Autodesk Fusion 360 part; units mm, degrees
note: some values were not read from the file. Set by a fixed rule: which sketch regions a step uses.
(part 4 of 59)
  spline S16 degree 5 poles (20.11, 33.4575) (20.11, 33.4576) (20.1102, 33.4577) (20.1104, 33.458) (20.1107, 33.4583) (20.1112, 33.4589) (20.1118, 33.4595) (20.1125, 33.4602) (20.1132, 33.461) (20.114, 33.4619) (20.1149, 33.4629) (20.1159, 33.4639) (20.1169, 33.4651) (20.118, 33.4663) (20.1192, 33.4675) (20.1204, 33.4689) (20.1217, 33.4704) (20.123, 33.4719) (20.1245, 33.4735) (20.126, 33.4752) (20.1275, 33.4769) (20.1291, 33.4787) (20.1308, 33.4806) (20.1325, 33.4826) (20.1343, 33.4847) (20.1361, 33.4868) (20.138, 33.489) (20.1399, 33.4912) (20.1419, 33.4936) (20.144, 33.496) (20.1461, 33.4984) (20.1482, 33.501) (20.1504, 33.5036) (20.1527, 33.5063) (20.155, 33.509) (20.1573, 33.5119) (20.1597, 33.5148) (20.1622, 33.5177) (20.1647, 33.5207) (20.1672, 33.5238) (20.1698, 33.527) (20.1724, 33.5302) (20.1751, 33.5335) (20.1778, 33.5368) (20.1806, 33.5403) (20.1834, 33.5437) (20.1862, 33.5473) (20.1891, 33.5509) (20.192, 33.5546) (20.195, 33.5583) (20.198, 33.5621) (20.201, 33.566) (20.2041, 33.5699) (20.2072, 33.5739) (20.2103, 33.5779) (20.2135, 33.582) (20.2167, 33.5862) (20.22, 33.5904) (20.2233, 33.5947) (20.2266, 33.599) (20.23, 33.6034) (20.2333, 33.6079) (20.2368, 33.6124) (20.2402, 33.617) (20.2437, 33.6216) (20.2472, 33.6263) (20.2508, 33.6311) (20.2544, 33.6359) (20.258, 33.6408) (20.2616, 33.6457) (20.2653, 33.6507) (20.269, 33.6557) (20.2727, 33.6608) (20.2765, 33.666) (20.2802, 33.6712) (20.2841, 33.6764) (20.2879, 33.6818) (20.2918, 33.6871) (20.2956, 33.6926) (20.2996, 33.6981) (20.3035, 33.7036) (20.3075, 33.7092) (20.3115, 33.7148) (20.3155, 33.7205) (20.3195, 33.7263) (20.3236, 33.7321) (20.3277, 33.738) (20.3318, 33.7439) (20.3359, 33.7498) (20.3401, 33.7559) (20.3442, 33.7619) (20.3484, 33.7681) (20.3527, 33.7742) (20.3569, 33.7805) (20.3612, 33.7867) (20.3655, 33.7931) (20.3698, 33.7995) (20.3741, 33.8059) (20.3784, 33.8124) (20.3828, 33.8189) (20.3872, 33.8255) (20.3916, 33.8321) (20.396, 33.8388) (20.4004, 33.8455) (20.4049, 33.8523) (20.4094, 33.8592) (20.4139, 33.8661) (20.4184, 33.873) (20.4229, 33.88) (20.4274, 33.887) (20.432, 33.8941) (20.4366, 33.9012) (20.4412, 33.9084) (20.4458, 33.9156) (20.4504, 33.9229) (20.455, 33.9302) (20.4597, 33.9376) (20.4644, 33.945) (20.469, 33.9525) (20.4737, 33.96) (20.4784, 33.9676) (20.4832, 33.9752) (20.4879, 33.9828) (20.4927, 33.9905) (20.4974, 33.9983) (20.5022, 34.0061) (20.507, 34.0139) (20.5118, 34.0218) (20.5166, 34.0297) (20.5214, 34.0377) (20.5263, 34.0458) (20.5311, 34.0538) (20.536, 34.0619) (20.5409, 34.0701) (20.5457, 34.0783) (20.5506, 34.0866) (20.5555, 34.0949) (20.5605, 34.1032) (20.5654, 34.1116) (20.5703, 34.1201) (20.5753, 34.1285) (20.5802, 34.1371) (20.5852, 34.1456) (20.5902, 34.1542) (20.5951, 34.1629) (20.6001, 34.1716) (20.6051, 34.1803) (20.6101, 34.1891) (20.6152, 34.198) (20.6202, 34.2068) (20.6252, 34.2158) (20.6303, 34.2247) (20.6353, 34.2337) (20.6404, 34.2428) (20.6454, 34.2519) (20.6505, 34.261) (20.6556, 34.2702) (20.6607, 34.2794) (20.6658, 34.2887) (20.6709, 34.298) (20.676, 34.3073) (20.6811, 34.3167) (20.6862, 34.3261) (20.6913, 34.3356) (20.6965, 34.3451) (20.7016, 34.3547) (20.7067, 34.3643) (20.7119, 34.3739) (20.717, 34.3836) (20.7222, 34.3933) (20.7274, 34.4031) (20.7325, 34.4129) (20.7377, 34.4228) (20.7429, 34.4326) (20.748, 34.4426) (20.7532, 34.4525) (20.7584, 34.4625) (20.7636, 34.4726) (20.7688, 34.4827) (20.774, 34.4928) (20.7792, 34.503) (20.7844, 34.5132) (20.7896, 34.5235) (20.7948, 34.5337) (20.8, 34.5441) (20.8052, 34.5544) (20.8105, 34.5649) (20.8157, 34.5753) (20.8209, 34.5858) (20.8261, 34.5963) (20.8313, 34.6069) (20.8366, 34.6175) (20.8418, 34.6281) (20.847, 34.6388) (20.8523, 34.6496) (20.8575, 34.6603) (20.8627, 34.6711) (20.868, 34.682) (20.8732, 34.6928) (20.8784, 34.7038) (20.8837, 34.7147) (20.8889, 34.7257) (20.8942, 34.7367) (20.8994, 34.7478) (20.9046, 34.7589) (20.9099, 34.7701) (20.9151, 34.7812) (20.9204, 34.7925) (20.9256, 34.8037) (20.9308, 34.815) (20.9361, 34.8264) (20.9413, 34.8377) (20.9466, 34.8491) (20.9518, 34.8606) (20.957, 34.8721) (20.9623, 34.8836) (20.9675, 34.8951) (20.9727, 34.9067) (20.978, 34.9184) (20.9832, 34.93) (20.9884, 34.9417) (20.9937, 34.9535) (20.9989, 34.9653) (21.0041, 34.9771) (21.0093, 34.9889) (21.0145, 35.0008) (21.0198, 35.0127) (21.025, 35.0247) (21.0302, 35.0367) (21.0354, 35.0487) (21.0406, 35.0608) (21.0458, 35.0729) (21.051, 35.085) (21.0562, 35.0972) (21.0614, 35.1094) (21.0666, 35.1217) (21.0718, 35.1339) (21.077, 35.1462) (21.0822, 35.1586) (21.0873, 35.171) (21.0925, 35.1834) (21.0967, 35.1934) (21.0998, 35.2009) (21.1018, 35.2059) (21.1029, 35.2084) knots 0 0 0 0 0 0 0.00416667 0.00833333 0.0125 0.01666667 0.02083333 0.025 0.02916667 0.03333333 0.0375 0.04166667 0.04583333 0.05 0.05416667 0.05833333 0.0625 0.06666667 0.07083333 0.075 0.07916667 0.08333333 0.0875 0.09166667 0.09583333 0.1 0.10416667 0.10833333 0.1125 0.11666667 0.12083333 0.125 0.12916667 0.13333333 0.1375 0.14166667 0.14583333 0.15 0.15416667 0.15833333 0.1625 0.16666667 0.17083333 0.175 0.17916667 0.18333333 0.1875 0.19166667 0.19583333 0.2 0.20416667 0.20833333 0.2125 0.21666667 0.22083333 0.225 0.22916667 0.23333333 0.2375 0.24166667 0.24583333 0.25 0.25416667 0.25833333 0.2625 0.26666667 0.27083333 0.275 0.27916667 0.28333333 0.2875 0.29166667 0.29583333 0.3 0.30416667 0.30833333 0.3125 0.31666667 0.32083333 0.325 0.32916667 0.33333333 0.3375 0.34166667 0.34583333 0.35 0.35416667 0.35833333 0.3625 0.36666667 0.37083333 0.375 0.37916667 0.38333333 0.3875 0.39166667 0.39583333 0.4 0.40416667 0.40833333 0.4125 0.41666667 0.42083333 0.425 0.42916667 0.43333333 0.4375 0.44166667 0.44583333 0.45 0.45416667 0.45833333 0.4625 0.46666667 0.47083333 0.475 0.47916667 0.48333333 0.4875 0.49166667 0.49583333 0.5 0.50416667 0.50833333 0.5125 0.51666667 0.52083333 0.525 0.52916667 0.53333333 0.5375 0.54166667 0.54583333 0.55 0.55416667 0.55833333 0.5625 0.56666667 0.57083333 0.575 0.57916667 0.58333333 0.5875 0.59166667 0.59583333 0.6 0.60416667 0.60833333 0.6125 0.61666667 0.62083333 0.625 0.62916667 0.63333333 0.6375 0.64166667 0.64583333 0.65 0.65416667 0.65833333 0.6625 0.66666667 0.67083333 0.675 0.67916667 0.68333333 0.6875 0.69166667 0.69583333 0.7 0.70416667 0.70833333 0.7125 0.71666667 0.72083333 0.725 0.72916667 0.73333333 0.7375 0.74166667 0.74583333 0.75 0.75416667 0.75833333 0.7625 0.76666667 0.77083333 0.775 0.77916667 0.78333333 0.7875 0.79166667 0.79583333 0.8 0.80416667 0.80833333 0.8125 0.81666667 0.82083333 0.825 0.82916667 0.83333333 0.8375 0.84166667 0.84583333 0.85 0.85416667 0.85833333 0.8625 0.86666667 0.87083333 0.875 0.87916667 0.88333333 0.8875 0.89166667 0.89583333 0.9 0.90416667 0.90833333 0.9125 0.91666667 0.92083333 0.925 0.92916667 0.93333333 0.9375 0.94166667 0.94583333 0.95 0.95416667 0.95833333 0.9625 0.96666667 0.97083333 0.975 0.97916667 0.98333333 0.9875 0.99166667 0.99583333 1 1 1 1 1 1
  spline S17 degree 5 poles (-17.8091, -10.4448) (-17.8092, -10.4448) (-17.8093, -10.445) (-17.8095, -10.4453) (-17.8098, -10.4457) (-17.8103, -10.4463) (-17.8108, -10.4469) (-17.8114, -10.4477) (-17.812, -10.4486) (-17.8127, -10.4496) (-17.8135, -10.4506) (-17.8144, -10.4518) (-17.8153, -10.453) (-17.8162, -10.4543) (-17.8172, -10.4557) (-17.8183, -10.4572) (-17.8195, -10.4588) (-17.8207, -10.4604) (-17.8219, -10.4622) (-17.8232, -10.464) (-17.8246, -10.4659) (-17.826, -10.4679) (-17.8274, -10.4699) (-17.8289, -10.4721) (-17.8305, -10.4743) (-17.8321, -10.4766) (-17.8337, -10.479) (-17.8354, -10.4814) (-17.8372, -10.484) (-17.8389, -10.4866) (-17.8408, -10.4893) (-17.8427, -10.492) (-17.8446, -10.4948) (-17.8465, -10.4978) (-17.8485, -10.5007) (-17.8506, -10.5038) (-17.8527, -10.5069) (-17.8548, -10.5101) (-17.857, -10.5134) (-17.8592, -10.5167) (-17.8614, -10.5201) (-17.8637, -10.5236) (-17.866, -10.5271) (-17.8683, -10.5308) (-17.8707, -10.5344) (-17.8731, -10.5382) (-17.8756, -10.542) (-17.8781, -10.5459) (-17.8806, -10.5499) (-17.8831, -10.5539) (-17.8857, -10.558) (-17.8883, -10.5621) (-17.891, -10.5664) (-17.8937, -10.5706) (-17.8964, -10.575) (-17.8991, -10.5794) (-17.9019, -10.5839) (-17.9047, -10.5884) (-17.9075, -10.593) (-17.9103, -10.5977) (-17.9132, -10.6024) (-17.9161, -10.6072) (-17.9191, -10.6121) (-17.922, -10.617) (-17.925, -10.622) (-17.928, -10.627) (-17.931, -10.6321) (-17.9341, -10.6373) (-17.9372, -10.6425) (-17.9403, -10.6478) (-17.9434, -10.6531) (-17.9466, -10.6585) (-17.9497, -10.664) (-17.9529, -10.6695) (-17.9562, -10.6751) (-17.9594, -10.6807) (-17.9627, -10.6864) (-17.9659, -10.6921) (-17.9692, -10.6979) (-17.9726, -10.7038) (-17.9759, -10.7097) (-17.9793, -10.7157) (-17.9826, -10.7217) (-17.986, -10.7278) (-17.9895, -10.734) (-17.9929, -10.7402) (-17.9963, -10.7464) (-17.9998, -10.7527) (-18.0033, -10.7591) (-18.0068, -10.7655) (-18.0103, -10.772) (-18.0139, -10.7785) (-18.0174, -10.7851) (-18.021, -10.7918) (-18.0246, -10.7984) (-18.0282, -10.8052) (-18.0318, -10.812) (-18.0354, -10.8188) (-18.039, -10.8257) (-18.0427, -10.8327) (-18.0464, -10.8397) (-18.0501, -10.8468) (-18.0538, -10.8539) (-18.0575, -10.861) (-18.0612, -10.8683) (-18.0649, -10.8755) (-18.0687, -10.8828) (-18.0724, -10.8902) (-18.0762, -10.8976) (-18.08, -10.9051) (-18.0838, -10.9126) (-18.0876, -10.9202) (-18.0914, -10.9278) (-18.0952, -10.9355) (-18.0991, -10.9432) (-18.1029, -10.951) (-18.1068, -10.9588) (-18.1106, -10.9666) (-18.1145, -10.9746) (-18.1184, -10.9825) (-18.1223, -10.9905) (-18.1262, -10.9986) (-18.1301, -11.0067) (-18.134, -11.0149) (-18.1379, -11.0231) (-18.1419, -11.0313) (-18.1458, -11.0396) (-18.1498, -11.048) (-18.1537, -11.0564) (-18.1577, -11.0648) (-18.1617, -11.0733) (-18.1657, -11.0818) (-18.1696, -11.0904) (-18.1736, -11.0991) (-18.1776, -11.1077) (-18.1816, -11.1165) (-18.1857, -11.1252) (-18.1897, -11.134) (-18.1937, -11.1429) (-18.1977, -11.1518) (-18.2018, -11.1607) (-18.2058, -11.1697) (-18.2098, -11.1788) (-18.2139, -11.1879) (-18.2179, -11.197) (-18.222, -11.2062) (-18.226, -11.2154) (-18.2301, -11.2247) (-18.2342, -11.234) (-18.2383, -11.2433) (-18.2423, -11.2527) (-18.2464, -11.2622) (-18.2505, -11.2716) (-18.2546, -11.2812) (-18.2587, -11.2907) (-18.2627, -11.3004) (-18.2668, -11.31) (-18.2709, -11.3197) (-18.275, -11.3295) (-18.2791, -11.3393) (-18.2832, -11.3491) (-18.2873, -11.359) (-18.2914, -11.3689) (-18.2955, -11.3788) (-18.2996, -11.3888) (-18.3038, -11.3989) (-18.3079, -11.409) (-18.312, -11.4191) (-18.3161, -11.4292) (-18.3202, -11.4395) (-18.3243, -11.4497) (-18.3284, -11.46) (-18.3325, -11.4703) (-18.3366, -11.4807) (-18.3408, -11.4911) (-18.3449, -11.5016) (-18.349, -11.5121) (-18.3531, -11.5226) (-18.3572, -11.5332) (-18.3613, -11.5438) (-18.3654, -11.5545) (-18.3695, -11.5652) (-18.3736, -11.5759) (-18.3777, -11.5867) (-18.3818, -11.5975) (-18.3859, -11.6084) (-18.39, -11.6193) (-18.3941, -11.6302) (-18.3982, -11.6412) (-18.4023, -11.6522) (-18.4064, -11.6633) (-18.4105, -11.6744) (-18.4146, -11.6855) (-18.4187, -11.6967) (-18.4228, -11.7079) (-18.4269, -11.7191) (-18.4309, -11.7304) (-18.435, -11.7417) (-18.4391, -11.7531) (-18.4431, -11.7645) (-18.4472, -11.776) (-18.4513, -11.7874) (-18.4553, -11.799) (-18.4594, -11.8105) (-18.4634, -11.8221) (-18.4675, -11.8337) (-18.4715, -11.8454) (-18.4756, -11.8571) (-18.4796, -11.8689) (-18.4836, -11.8806) (-18.4877, -11.8925) (-18.4917, -11.9043) (-18.4957, -11.9162) (-18.4997, -11.9281) (-18.5037, -11.9401) (-18.5077, -11.9521) (-18.5117, -11.9642) (-18.5157, -11.9762) (-18.5197, -11.9884) (-18.5237, -12.0005) (-18.5277, -12.0127) (-18.5316, -12.0249) (-18.5356, -12.0372) (-18.5395, -12.0495) (-18.5435, -12.0618) (-18.5475, -12.0742) (-18.5514, -12.0866) (-18.5553, -12.099) (-18.5593, -12.1115) (-18.5632, -12.124) (-18.5671, -12.1365) (-18.571, -12.1491) (-18.5749, -12.1617) (-18.5788, -12.1744) (-18.5827, -12.1871) (-18.5866, -12.1998) (-18.5905, -12.2125) (-18.5943, -12.2253) (-18.5982, -12.2382) (-18.6021, -12.251) (-18.6059, -12.2639) (-18.609, -12.2743) (-18.6113, -12.282) (-18.6128, -12.2872) (-18.6136, -12.2898) knots 0 0 0 0 0 0 0.00416667 0.00833333 0.0125 0.01666667 0.02083333 0.025 0.02916667 0.03333333 0.0375 0.04166667 0.04583333 0.05 0.05416667 0.05833333 0.0625 0.06666667 0.07083333 0.075 0.07916667 0.08333333 0.0875 0.09166667 0.09583333 0.1 0.10416667 0.10833333 0.1125 0.11666667 0.12083333 0.125 0.12916667 0.13333333 0.1375 0.14166667 0.14583333 0.15 0.15416667 0.15833333 0.1625 0.16666667 0.17083333 0.175 0.17916667 0.18333333 0.1875 0.19166667 0.19583333 0.2 0.20416667 0.20833333 0.2125 0.21666667 0.22083333 0.225 0.22916667 0.23333333 0.2375 0.24166667 0.24583333 0.25 0.25416667 0.25833333 0.2625 0.26666667 0.27083333 0.275 0.27916667 0.28333333 0.2875 0.29166667 0.29583333 0.3 0.30416667 0.30833333 0.3125 0.31666667 0.32083333 0.325 0.32916667 0.33333333 0.3375 0.34166667 0.34583333 0.35 0.35416667 0.35833333 0.3625 0.36666667 0.37083333 0.375 0.37916667 0.38333333 0.3875 0.39166667 0.39583333 0.4 0.40416667 0.40833333 0.4125 0.41666667 0.42083333 0.425 0.42916667 0.43333333 0.4375 0.44166667 0.44583333 0.45 0.45416667 0.45833333 0.4625 0.46666667 0.47083333 0.475 0.47916667 0.48333333 0.4875 0.49166667 0.49583333 0.5 0.50416667 0.50833333 0.5125 0.51666667 0.52083333 0.525 0.52916667 0.53333333 0.5375 0.54166667 0.54583333 0.55 0.55416667 0.55833333 0.5625 0.56666667 0.57083333 0.575 0.57916667 0.58333333 0.5875 0.59166667 0.59583333 0.6 0.60416667 0.60833333 0.6125 0.61666667 0.62083333 0.625 0.62916667 0.63333333 0.6375 0.64166667 0.64583333 0.65 0.65416667 0.65833333 0.6625 0.66666667 0.67083333 0.675 0.67916667 0.68333333 0.6875 0.69166667 0.69583333 0.7 0.70416667 0.70833333 0.7125 0.71666667 0.72083333 0.725 0.72916667 0.73333333 0.7375 0.74166667 0.74583333 0.75 0.75416667 0.75833333 0.7625 0.76666667 0.77083333 0.775 0.77916667 0.78333333 0.7875 0.79166667 0.79583333 0.8 0.80416667 0.80833333 0.8125 0.81666667 0.82083333 0.825 0.82916667 0.83333333 0.8375 0.84166667 0.84583333 0.85 0.85416667 0.85833333 0.8625 0.86666667 0.87083333 0.875 0.87916667 0.88333333 0.8875 0.89166667 0.89583333 0.9 0.90416667 0.90833333 0.9125 0.91666667 0.92083333 0.925 0.92916667 0.93333333 0.9375 0.94166667 0.94583333 0.95 0.95416667 0.95833333 0.9625 0.96666667 0.97083333 0.975 0.97916667 0.98333333 0.9875 0.99166667 0.99583333 1 1 1 1 1 1
  arc A27 (-18.6136, -12.2898) -> (-17.8246, -12.863) centre (0, 12.5) ccw
  line L63 (-28.2039, 19.4368) -> (-28.2047, 19.437)
  line L64 (-25.3417, -1.078) -> (-25.6012, -1.2171)
  spline S18 degree 5 poles (-29.6298, 21.6146) (-29.6276, 21.6129) (-29.6234, 21.6096) (-29.6169, 21.6047) (-29.6084, 21.5981) (-29.5977, 21.59) (-29.587, 21.5818) (-29.5763, 21.5737) (-29.5657, 21.5657) (-29.555, 21.5576) (-29.5444, 21.5496) (-29.5338, 21.5416) (-29.5232, 21.5337) (-29.5127, 21.5258) (-29.5021, 21.5179) (-29.4915, 21.5101) (-29.481, 21.5022) (-29.4705, 21.4945) (-29.46, 21.4867) (-29.4495, 21.479) (-29.4391, 21.4713) (-29.4286, 21.4637) (-29.4182, 21.456) (-29.4078, 21.4485) (-29.3974, 21.4409) (-29.387, 21.4334) (-29.3766, 21.4259) (-29.3663, 21.4184) (-29.356, 21.411) (-29.3457, 21.4036) (-29.3354, 21.3963) (-29.3251, 21.3889) (-29.3148, 21.3816) (-29.3046, 21.3744) (-29.2944, 21.3671) (-29.2842, 21.36) (-29.274, 21.3528) (-29.2638, 21.3457) (-29.2537, 21.3386) (-29.2435, 21.3315) (-29.2334, 21.3245) (-29.2233, 21.3175) (-29.2132, 21.3105) (-29.2032, 21.3036) (-29.1932, 21.2967) (-29.1831, 21.2898) (-29.1731, 21.283) (-29.1632, 21.2762) (-29.1532, 21.2694) (-29.1433, 21.2626) (-29.1334, 21.2559) (-29.1235, 21.2493) (-29.1136, 21.2426) (-29.1037, 21.236) (-29.0939, 21.2295) (-29.0841, 21.2229) (-29.0743, 21.2164) (-29.0646, 21.2099) (-29.0548, 21.2035) (-29.0451, 21.1971) (-29.0354, 21.1907) (-29.0257, 21.1844) (-29.016, 21.1781) (-29.0064, 21.1718) (-28.9968, 21.1656) (-28.9872, 21.1593) (-28.9776, 21.1532) (-28.9681, 21.147) (-28.9586, 21.1409) (-28.9491, 21.1348) (-28.9396, 21.1288) (-28.9302, 21.1228) (-28.9207, 21.1168) (-28.9113, 21.1109) (-28.902, 21.105) (-28.8926, 21.0991) (-28.8833, 21.0932) (-28.874, 21.0874) (-28.8647, 21.0817) (-28.8555, 21.0759) (-28.8462, 21.0702) (-28.837, 21.0645) (-28.8279, 21.0589) (-28.8187, 21.0533) (-28.8096, 21.0477) (-28.8005, 21.0422) (-28.7914, 21.0367) (-28.7824, 21.0312) (-28.7734, 21.0257) (-28.7644, 21.0203) (-28.7554, 21.015) (-28.7465, 21.0096) (-28.7376, 21.0043) (-28.7287, 20.999) (-28.7199, 20.9938) (-28.711, 20.9886) (-28.7022, 20.9834) (-28.6935, 20.9783) (-28.6847, 20.9732) (-28.676, 20.9681) (-28.6674, 20.963) (-28.6587, 20.958) (-28.6501, 20.9531) (-28.6415, 20.9481) (-28.633, 20.9432) (-28.6244, 20.9384) (-28.616, 20.9335) (-28.6075, 20.9287) (-28.5991, 20.9239) (-28.5907, 20.9192) (-28.5823, 20.9145) (-28.574, 20.9098) (-28.5657, 20.9052) (-28.5574, 20.9006) (-28.5491, 20.896) (-28.5409, 20.8915) (-28.5328, 20.887) (-28.5246, 20.8825) (-28.5165, 20.8781) (-28.5085, 20.8737) (-28.5004, 20.8693) (-28.4924, 20.865) (-28.4845, 20.8607) (-28.4765, 20.8565) (-28.4686, 20.8522) (-28.4608, 20.848) (-28.4529, 20.8439) (-28.4452, 20.8398) (-28.4374, 20.8357) (-28.4297, 20.8316) (-28.422, 20.8276) (-28.4144, 20.8236) (-28.4068, 20.8196) (-28.3992, 20.8157) (-28.3917, 20.8118) (-28.3842, 20.808) (-28.3767, 20.8042) (-28.3693, 20.8004) (-28.3619, 20.7966) (-28.3546, 20.7929) (-28.3473, 20.7892) (-28.3401, 20.7856) (-28.3329, 20.782) (-28.3257, 20.7784) (-28.3186, 20.7748) (-28.3115, 20.7713) (-28.3044, 20.7678) (-28.2974, 20.7644) (-28.2905, 20.761) (-28.2835, 20.7576) (-28.2767, 20.7543) (-28.2698, 20.751) (-28.263, 20.7477) (-28.2563, 20.7445) (-28.2496, 20.7412) (-28.2429, 20.7381) (-28.2363, 20.7349) (-28.2298, 20.7318) (-28.2233, 20.7288) (-28.2168, 20.7257) (-28.2104, 20.7227) (-28.204, 20.7198) (-28.1977, 20.7169) (-28.1914, 20.714) (-28.1851, 20.7111) (-28.179, 20.7083) (-28.1728, 20.7055) (-28.1667, 20.7027) (-28.1607, 20.7) (-28.1547, 20.6973) (-28.1488, 20.6947) (-28.1429, 20.692) (-28.1371, 20.6895) (-28.1313, 20.6869) (-28.1256, 20.6844) (-28.1199, 20.6819) (-28.1143, 20.6795) (-28.1087, 20.677) (-28.1032, 20.6747) (-28.0978, 20.6723) (-28.0924, 20.67) (-28.087, 20.6677) (-28.0818, 20.6655) (-28.0765, 20.6633) (-28.0714, 20.6611) (-28.0663, 20.659) (-28.0612, 20.6569) (-28.0562, 20.6548) (-28.0513, 20.6528) (-28.0464, 20.6508) (-28.0416, 20.6488) (-28.0369, 20.6469) (-28.0322, 20.645) (-28.0276, 20.6432) (-28.023, 20.6413) (-28.0185, 20.6395) (-28.0141, 20.6378) (-28.0097, 20.6361) (-28.0054, 20.6344) (-28.0012, 20.6327) (-27.997, 20.6311) (-27.9929, 20.6295) (-27.9889, 20.628) (-27.9849, 20.6265) (-27.9811, 20.625) (-27.9772, 20.6236) (-27.9735, 20.6222) (-27.9698, 20.6208) (-27.9662, 20.6194) (-27.9627, 20.6181) (-27.9593, 20.6169) (-27.9559, 20.6156) (-27.9526, 20.6144) (-27.9494, 20.6133) (-27.9462, 20.6121) (-27.9432, 20.6111) (-27.9402, 20.61) (-27.9373, 20.609) (-27.9345, 20.608) (-27.9318, 20.607) (-27.9291, 20.6061) (-27.9265, 20.6052) (-27.9241, 20.6044) (-27.9217, 20.6036) (-27.9194, 20.6028) (-27.9172, 20.602) (-27.915, 20.6013) (-27.913, 20.6007) (-27.9111, 20.6) (-27.9092, 20.5994) (-27.9075, 20.5988) (-27.9058, 20.5983) (-27.9043, 20.5978) (-27.9028, 20.5973) (-27.9015, 20.5969) (-27.9002, 20.5965) (-27.8991, 20.5962) (-27.898, 20.5958) (-27.8971, 20.5956) (-27.8963, 20.5953) (-27.8956, 20.5951) (-27.8951, 20.5949) (-27.8948, 20.5948) (-27.8946, 20.5948) (-27.8945, 20.5948) knots -1 -1 -1 -1 -1 -1 -0.99583333 -0.99166667 -0.9875 -0.98333333 -0.97916667 -0.975 -0.97083333 -0.96666667 -0.9625 -0.95833333 -0.95416667 -0.95 -0.94583333 -0.94166667 -0.9375 -0.93333333 -0.92916667 -0.925 -0.92083333 -0.91666667 -0.9125 -0.90833333 -0.90416667 -0.9 -0.89583333 -0.89166667 -0.8875 -0.88333333 -0.87916667 -0.875 -0.87083333 -0.86666667 -0.8625 -0.85833333 -0.85416667 -0.85 -0.84583333 -0.84166667 -0.8375 -0.83333333 -0.82916667 -0.825 -0.82083333 -0.81666667 -0.8125 -0.80833333 -0.80416667 -0.8 -0.79583333 -0.79166667 -0.7875 -0.78333333 -0.77916667 -0.775 -0.77083333 -0.76666667 -0.7625 -0.75833333 -0.75416667 -0.75 -0.74583333 -0.74166667 -0.7375 -0.73333333 -0.72916667 -0.725 -0.72083333 -0.71666667 -0.7125 -0.70833333 -0.70416667 -0.7 -0.69583333 -0.69166667 -0.6875 -0.68333333 -0.67916667 -0.675 -0.67083333 -0.66666667 -0.6625 -0.65833333 -0.65416667 -0.65 -0.64583333 -0.64166667 -0.6375 -0.63333333 -0.62916667 -0.625 -0.62083333 -0.61666667 -0.6125 -0.60833333 -0.60416667 -0.6 -0.59583333 -0.59166667 -0.5875 -0.58333333 -0.57916667 -0.575 -0.57083333 -0.56666667 -0.5625 -0.55833333 -0.55416667 -0.55 -0.54583333 -0.54166667 -0.5375 -0.53333333 -0.52916667 -0.525 -0.52083333 -0.51666667 -0.5125 -0.50833333 -0.50416667 -0.5 -0.49583333 -0.49166667 -0.4875 -0.48333333 -0.47916667 -0.475 -0.47083333 -0.46666667 -0.4625 -0.45833333 -0.45416667 -0.45 -0.44583333 -0.44166667 -0.4375 -0.43333333 -0.42916667 -0.425 -0.42083333 -0.41666667 -0.4125 -0.40833333 -0.40416667 -0.4 -0.39583333 -0.39166667 -0.3875 -0.38333333 -0.37916667 -0.375 -0.37083333 -0.36666667 -0.3625 -0.35833333 -0.35416667 -0.35 -0.34583333 -0.34166667 -0.3375 -0.33333333 -0.32916667 -0.325 -0.32083333 -0.31666667 -0.3125 -0.30833333 -0.30416667 -0.3 -0.29583333 -0.29166667 -0.2875 -0.28333333 -0.27916667 -0.275 -0.27083333 -0.26666667 -0.2625 -0.25833333 -0.25416667 -0.25 -0.24583333 -0.24166667 -0.2375 -0.23333333 -0.22916667 -0.225 -0.22083333 -0.21666667 -0.2125 -0.20833333 -0.20416667 -0.2 -0.19583333 -0.19166667 -0.1875 -0.18333333 -0.17916667 -0.175 -0.17083333 -0.16666667 -0.1625 -0.15833333 -0.15416667 -0.15 -0.14583333 -0.14166667 -0.1375 -0.13333333 -0.12916667 -0.125 -0.12083333 -0.11666667 -0.1125 -0.10833333 -0.10416667 -0.1 -0.09583333 -0.09166667 -0.0875 -0.08333333 -0.07916667 -0.075 -0.07083333 -0.06666667 -0.0625 -0.05833333 -0.05416667 -0.05 -0.04583333 -0.04166667 -0.0375 -0.03333333 -0.02916667 -0.025 -0.02083333 -0.01666667 -0.0125 -0.00833333 -0.00416667 0 0 0 0 0 0
  spline S19 degree 5 poles (-26.8955, 1.5338) (-26.8956, 1.5338) (-26.8958, 1.5337) (-26.8961, 1.5336) (-26.8966, 1.5334) (-26.8973, 1.5331) (-26.8981, 1.5328) (-26.899, 1.5324) (-26.9, 1.5319) (-26.9011, 1.5315) (-26.9023, 1.5309) (-26.9036, 1.5304) (-26.905, 1.5298) (-26.9065, 1.5291) (-26.908, 1.5284) (-26.9097, 1.5276) (-26.9115, 1.5269) (-26.9134, 1.526) (-26.9153, 1.5251) (-26.9173, 1.5242) (-26.9195, 1.5232) (-26.9217, 1.5222) (-26.924, 1.5212) (-26.9263, 1.5201) (-26.9288, 1.5189) (-26.9313, 1.5177) (-26.9339, 1.5165) (-26.9366, 1.5152) (-26.9394, 1.5139) (-26.9423, 1.5125) (-26.9452, 1.5111) (-26.9482, 1.5097) (-26.9513, 1.5082) (-26.9544, 1.5066) (-26.9577, 1.5051) (-26.961, 1.5034) (-26.9643, 1.5018) (-26.9678, 1.5001) (-26.9713, 1.4983) (-26.9748, 1.4965) (-26.9785, 1.4947) (-26.9822, 1.4928) (-26.986, 1.4909) (-26.9898, 1.4889) (-26.9937, 1.4869) (-26.9977, 1.4849) (-27.0017, 1.4828) (-27.0058, 1.4807) (-27.01, 1.4785) (-27.0142, 1.4763) (-27.0185, 1.4741) (-27.0228, 1.4718) (-27.0272, 1.4694) (-27.0317, 1.4671) (-27.0362, 1.4647) (-27.0408, 1.4622) (-27.0454, 1.4597) (-27.0501, 1.4572) (-27.0549, 1.4546) (-27.0597, 1.452) (-27.0645, 1.4493) (-27.0694, 1.4466) (-27.0744, 1.4439) (-27.0794, 1.4411) (-27.0845, 1.4383) (-27.0896, 1.4354) (-27.0948, 1.4325) (-27.1, 1.4296) (-27.1053, 1.4266) (-27.1106, 1.4236) (-27.116, 1.4205) (-27.1214, 1.4174) (-27.1269, 1.4143) (-27.1324, 1.4111) (-27.138, 1.4079) (-27.1436, 1.4046) (-27.1493, 1.4013) (-27.155, 1.398) (-27.1608, 1.3946) (-27.1666, 1.3912) (-27.1725, 1.3877) (-27.1784, 1.3842) (-27.1843, 1.3807) (-27.1903, 1.3771) (-27.1963, 1.3735) (-27.2024, 1.3699) (-27.2085, 1.3662) (-27.2147, 1.3624) (-27.2209, 1.3587) (-27.2271, 1.3549) (-27.2334, 1.351) (-27.2397, 1.3471) (-27.2461, 1.3432) (-27.2525, 1.3392) (-27.259, 1.3352) (-27.2654, 1.3312) (-27.272, 1.3271) (-27.2785, 1.323) (-27.2851, 1.3188) (-27.2918, 1.3146) (-27.2985, 1.3104) (-27.3052, 1.3061) (-27.3119, 1.3018) (-27.3187, 1.2975) (-27.3256, 1.2931) (-27.3324, 1.2887) (-27.3393, 1.2842) (-27.3463, 1.2797) (-27.3533, 1.2752) (-27.3603, 1.2706) (-27.3673, 1.266) (-27.3744, 1.2613) (-27.3815, 1.2566) (-27.3887, 1.2519) (-27.3958, 1.2471) (-27.4031, 1.2423) (-27.4103, 1.2375) (-27.4176, 1.2326) (-27.4249, 1.2277) (-27.4323, 1.2227) (-27.4396, 1.2177) (-27.447, 1.2127) (-27.4545, 1.2076) (-27.462, 1.2025) (-27.4695, 1.1974) (-27.477, 1.1922) (-27.4846, 1.187) (-27.4922, 1.1817) (-27.4998, 1.1765) (-27.5074, 1.1711) (-27.5151, 1.1658) (-27.5228, 1.1604) (-27.5306, 1.1549) (-27.5384, 1.1494) (-27.5462, 1.1439) (-27.554, 1.1384) (-27.5618, 1.1328) (-27.5697, 1.1272) (-27.5776, 1.1215) (-27.5856, 1.1158) (-27.5936, 1.1101) (-27.6015, 1.1043) (-27.6096, 1.0985) (-27.6176, 1.0926) (-27.6257, 1.0868) (-27.6338, 1.0808) (-27.6419, 1.0749) (-27.6501, 1.0689) (-27.6582, 1.0629) (-27.6665, 1.0568) (-27.6747, 1.0507) (-27.6829, 1.0446) (-27.6912, 1.0384) (-27.6995, 1.0322) (-27.7078, 1.0259) (-27.7162, 1.0197) (-27.7246, 1.0133) (-27.733, 1.007) (-27.7414, 1.0006) (-27.7498, 0.9942) (-27.7583, 0.9877) (-27.7668, 0.9812) (-27.7753, 0.9747) (-27.7838, 0.9681) (-27.7924, 0.9615) (-27.801, 0.9548) (-27.8096, 0.9482) (-27.8182, 0.9415) (-27.8268, 0.9347) (-27.8355, 0.9279) (-27.8442, 0.9211) (-27.8529, 0.9142) (-27.8616, 0.9073) (-27.8704, 0.9004) (-27.8791, 0.8935) (-27.8879, 0.8865) (-27.8967, 0.8794) (-27.9055, 0.8724) (-27.9144, 0.8652) (-27.9233, 0.8581) (-27.9322, 0.8509) (-27.9411, 0.8437) (-27.95, 0.8365) (-27.9589, 0.8292) (-27.9679, 0.8219) (-27.9769, 0.8145) (-27.9859, 0.8071) (-27.9949, 0.7997) (-28.0039, 0.7922) (-28.013, 0.7847) (-28.0221, 0.7772) (-28.0312, 0.7697) (-28.0403, 0.7621) (-28.0494, 0.7544) (-28.0585, 0.7468) (-28.0677, 0.7391) (-28.0769, 0.7313) (-28.0861, 0.7235) (-28.0953, 0.7157) (-28.1045, 0.7079) (-28.1137, 0.7) (-28.123, 0.6921) (-28.1323, 0.6842) (-28.1416, 0.6762) (-28.1509, 0.6682) (-28.1602, 0.6601) (-28.1695, 0.652) (-28.1789, 0.6439) (-28.1882, 0.6357) (-28.1976, 0.6276) (-28.207, 0.6193) (-28.2164, 0.6111) (-28.2259, 0.6028) (-28.2353, 0.5945) (-28.2447, 0.5861) (-28.2542, 0.5777) (-28.2637, 0.5693) (-28.2732, 0.5608) (-28.2827, 0.5523) (-28.2922, 0.5438) (-28.3018, 0.5352) (-28.3113, 0.5266) (-28.3209, 0.518) (-28.3305, 0.5093) (-28.34, 0.5006) (-28.3496, 0.4919) (-28.3593, 0.4831) (-28.3689, 0.4743) (-28.3785, 0.4655) (-28.3882, 0.4566) (-28.3978, 0.4477) (-28.4075, 0.4387) (-28.4172, 0.4298) (-28.4269, 0.4208) (-28.4366, 0.4117) (-28.4464, 0.4027) (-28.4561, 0.3935) (-28.4658, 0.3844) (-28.4756, 0.3752) (-28.4854, 0.366) (-28.4951, 0.3568) (-28.503, 0.3494) (-28.5089, 0.3438) (-28.5128, 0.34) (-28.5147, 0.3382) knots 0 0 0 0 0 0 0.00416667 0.00833333 0.0125 0.01666667 0.02083333 0.025 0.02916667 0.03333333 0.0375 0.04166667 0.04583333 0.05 0.05416667 0.05833333 0.0625 0.06666667 0.07083333 0.075 0.07916667 0.08333333 0.0875 0.09166667 0.09583333 0.1 0.10416667 0.10833333 0.1125 0.11666667 0.12083333 0.125 0.12916667 0.13333333 0.1375 0.14166667 0.14583333 0.15 0.15416667 0.15833333 0.1625 0.16666667 0.17083333 0.175 0.17916667 0.18333333 0.1875 0.19166667 0.19583333 0.2 0.20416667 0.20833333 0.2125 0.21666667 0.22083333 0.225 0.22916667 0.23333333 0.2375 0.24166667 0.24583333 0.25 0.25416667 0.25833333 0.2625 0.26666667 0.27083333 0.275 0.27916667 0.28333333 0.2875 0.29166667 0.29583333 0.3 0.30416667 0.30833333 0.3125 0.31666667 0.32083333 0.325 0.32916667 0.33333333 0.3375 0.34166667 0.34583333 0.35 0.35416667 0.35833333 0.3625 0.36666667 0.37083333 0.375 0.37916667 0.38333333 0.3875 0.39166667 0.39583333 0.4 0.40416667 0.40833333 0.4125 0.41666667 0.42083333 0.425 0.42916667 0.43333333 0.4375 0.44166667 0.44583333 0.45 0.45416667 0.45833333 0.4625 0.46666667 0.47083333 0.475 0.47916667 0.48333333 0.4875 0.49166667 0.49583333 0.5 0.50416667 0.50833333 0.5125 0.51666667 0.52083333 0.525 0.52916667 0.53333333 0.5375 0.54166667 0.54583333 0.55 0.55416667 0.55833333 0.5625 0.56666667 0.57083333 0.575 0.57916667 0.58333333 0.5875 0.59166667 0.59583333 0.6 0.60416667 0.60833333 0.6125 0.61666667 0.62083333 0.625 0.62916667 0.63333333 0.6375 0.64166667 0.64583333 0.65 0.65416667 0.65833333 0.6625 0.66666667 0.67083333 0.675 0.67916667 0.68333333 0.6875 0.69166667 0.69583333 0.7 0.70416667 0.70833333 0.7125 0.71666667 0.72083333 0.725 0.72916667 0.73333333 0.7375 0.74166667 0.74583333 0.75 0.75416667 0.75833333 0.7625 0.76666667 0.77083333 0.775 0.77916667 0.78333333 0.7875 0.79166667 0.79583333 0.8 0.80416667 0.80833333 0.8125 0.81666667 0.82083333 0.825 0.82916667 0.83333333 0.8375 0.84166667 0.84583333 0.85 0.85416667 0.85833333 0.8625 0.86666667 0.87083333 0.875 0.87916667 0.88333333 0.8875 0.89166667 0.89583333 0.9 0.90416667 0.90833333 0.9125 0.91666667 0.92083333 0.925 0.92916667 0.93333333 0.9375 0.94166667 0.94583333 0.95 0.95416667 0.95833333 0.9625 0.96666667 0.97083333 0.975 0.97916667 0.98333333 0.9875 0.99166667 0.99583333 1 1 1 1 1 1
  spline S20 degree 5 poles (20.3781, 35.8609) (20.3757, 35.8596) (20.371, 35.8571) (20.3639, 35.8532) (20.3544, 35.848) (20.3426, 35.8416) (20.3308, 35.8351) (20.319, 35.8287) (20.3073, 35.8222) (20.2957, 35.8158) (20.284, 35.8094) (20.2724, 35.8029) (20.2609, 35.7965) (20.2493, 35.79) (20.2379, 35.7836) (20.2264, 35.7771) (20.215, 35.7707) (20.2036, 35.7643) (20.1922, 35.7578) (20.1809, 35.7514) (20.1697, 35.745) (20.1584, 35.7385) (20.1472, 35.7321) (20.136, 35.7257) (20.1249, 35.7193) (20.1138, 35.7128) (20.1028, 35.7064) (20.0917, 35.7) (20.0808, 35.6936) (20.0698, 35.6872) (20.0589, 35.6807) (20.048, 35.6743) (20.0372, 35.6679) (20.0264, 35.6615) (20.0156, 35.6551) (20.0049, 35.6487) (19.9942, 35.6423) (19.9836, 35.636) (19.973, 35.6296) (19.9624, 35.6232) (19.9518, 35.6168) (19.9413, 35.6104) (19.9309, 35.6041) (19.9205, 35.5977) (19.9101, 35.5914) (19.8997, 35.585) (19.8894, 35.5786) (19.8791, 35.5723) (19.8689, 35.566) (19.8587, 35.5596) (19.8486, 35.5533) (19.8384, 35.547) (19.8284, 35.5406) (19.8183, 35.5343) (19.8083, 35.528) (19.7984, 35.5217) (19.7884, 35.5154) (19.7785, 35.5091) (19.7687, 35.5029) (19.7589, 35.4966) (19.7491, 35.4903) (19.7394, 35.484) (19.7297, 35.4778) (19.72, 35.4715) (19.7104, 35.4653) (19.7009, 35.4591) (19.6913, 35.4528) (19.6818, 35.4466) (19.6724, 35.4404) (19.663, 35.4342) (19.6536, 35.428) (19.6443, 35.4218) (19.635, 35.4156) (19.6257, 35.4095) (19.6165, 35.4033) (19.6073, 35.3971) (19.5982, 35.391) (19.5891, 35.3849) (19.5801, 35.3787) (19.5711, 35.3726) (19.5621, 35.3665) (19.5532, 35.3604) (19.5443, 35.3543) (19.5354, 35.3483) (19.5266, 35.3422) (19.5179, 35.3361) (19.5091, 35.3301) (19.5005, 35.3241) (19.4918, 35.318) (19.4832, 35.312) (19.4747, 35.306) (19.4662, 35.3) (19.4577, 35.2941) (19.4493, 35.2881) (19.4409, 35.2822) (19.4325, 35.2762) (19.4242, 35.2703) (19.416, 35.2644) (19.4078, 35.2585) (19.3996, 35.2526) (19.3914, 35.2467) (19.3834, 35.2408) (19.3753, 35.235) (19.3673, 35.2292) (19.3593, 35.2233) (19.3514, 35.2175) (19.3436, 35.2118) (19.3357, 35.206) (19.3279, 35.2002) (19.3202, 35.1945) (19.3125, 35.1887) (19.3048, 35.183) (19.2972, 35.1773) (19.2897, 35.1716) (19.2821, 35.166) (19.2747, 35.1603) (19.2672, 35.1547) (19.2598, 35.1491) (19.2525, 35.1435) (19.2452, 35.1379) (19.2379, 35.1323) (19.2307, 35.1268) (19.2236, 35.1212) (19.2165, 35.1157) (19.2094, 35.1102) (19.2024, 35.1048) (19.1954, 35.0993) (19.1884, 35.0939) (19.1815, 35.0884) (19.1747, 35.083) (19.1679, 35.0777) (19.1611, 35.0723) (19.1544, 35.067) (19.1478, 35.0617) (19.1412, 35.0564) (19.1346, 35.0511) (19.1281, 35.0458) (19.1216, 35.0406) (19.1152, 35.0354) (19.1088, 35.0302) (19.1025, 35.025) (19.0962, 35.0199) (19.09, 35.0148) (19.0838, 35.0097) (19.0776, 35.0046) (19.0715, 34.9996) (19.0655, 34.9945) (19.0595, 34.9895) (19.0536, 34.9846) (19.0477, 34.9796) (19.0418, 34.9747) (19.036, 34.9698) (19.0303, 34.9649) (19.0246, 34.9601) (19.0189, 34.9553) (19.0133, 34.9505) (19.0077, 34.9457) (19.0022, 34.941) (18.9968, 34.9363) (18.9914, 34.9316) (18.986, 34.927) (18.9807, 34.9223) (18.9755, 34.9177) (18.9703, 34.9132) (18.9651, 34.9087) (18.96, 34.9042) (18.955, 34.8997) (18.95, 34.8953) (18.9451, 34.8909) (18.9402, 34.8865) (18.9353, 34.8821) (18.9306, 34.8778) (18.9258, 34.8736) (18.9211, 34.8693) (18.9165, 34.8651) (18.9119, 34.8609) (18.9074, 34.8568) (18.903, 34.8527) (18.8986, 34.8486) (18.8942, 34.8446) (18.8899, 34.8406) (18.8856, 34.8367) (18.8814, 34.8328) (18.8773, 34.8289) (18.8732, 34.825) (18.8692, 34.8212) (18.8652, 34.8175) (18.8613, 34.8138) (18.8574, 34.8101) (18.8536, 34.8065) (18.8499, 34.8029) (18.8462, 34.7993) (18.8426, 34.7958) (18.839, 34.7923) (18.8355, 34.7889) (18.832, 34.7855) (18.8286, 34.7822) (18.8252, 34.7789) (18.822, 34.7757) (18.8187, 34.7725) (18.8156, 34.7693) (18.8124, 34.7662) (18.8094, 34.7632) (18.8064, 34.7602) (18.8035, 34.7572) (18.8006, 34.7543) (18.7978, 34.7515) (18.7951, 34.7487) (18.7924, 34.7459) (18.7897, 34.7433) (18.7872, 34.7406) (18.7847, 34.738) (18.7823, 34.7355) (18.7799, 34.7331) (18.7776, 34.7307) (18.7753, 34.7283) (18.7732, 34.726) (18.771, 34.7238) (18.769, 34.7216) (18.767, 34.7195) (18.7651, 34.7175) (18.7632, 34.7155) (18.7615, 34.7136) (18.7597, 34.7117) (18.7581, 34.7099) (18.7565, 34.7082) (18.755, 34.7066) (18.7536, 34.705) (18.7522, 34.7035) (18.7509, 34.702) (18.7497, 34.7007) (18.7485, 34.6994) (18.7474, 34.6982) (18.7464, 34.697) (18.7455, 34.696) (18.7446, 34.695) (18.7438, 34.6941) (18.7431, 34.6933) (18.7424, 34.6925) (18.7419, 34.6919) (18.7414, 34.6913) (18.741, 34.6909) (18.7408, 34.6907) (18.7407, 34.6905) (18.7406, 34.6904) knots -1 -1 -1 -1 -1 -1 -0.99583333 -0.99166667 -0.9875 -0.98333333 -0.97916667 -0.975 -0.97083333 -0.96666667 -0.9625 -0.95833333 -0.95416667 -0.95 -0.94583333 -0.94166667 -0.9375 -0.93333333 -0.92916667 -0.925 -0.92083333 -0.91666667 -0.9125 -0.90833333 -0.90416667 -0.9 -0.89583333 -0.89166667 -0.8875 -0.88333333 -0.87916667 -0.875 -0.87083333 -0.86666667 -0.8625 -0.85833333 -0.85416667 -0.85 -0.84583333 -0.84166667 -0.8375 -0.83333333 -0.82916667 -0.825 -0.82083333 -0.81666667 -0.8125 -0.80833333 -0.80416667 -0.8 -0.79583333 -0.79166667 -0.7875 -0.78333333 -0.77916667 -0.775 -0.77083333 -0.76666667 -0.7625 -0.75833333 -0.75416667 -0.75 -0.74583333 -0.74166667 -0.7375 -0.73333333 -0.72916667 -0.725 -0.72083333 -0.71666667 -0.7125 -0.70833333 -0.70416667 -0.7 -0.69583333 -0.69166667 -0.6875 -0.68333333 -0.67916667 -0.675 -0.67083333 -0.66666667 -0.6625 -0.65833333 -0.65416667 -0.65 -0.64583333 -0.64166667 -0.6375 -0.63333333 -0.62916667 -0.625 -0.62083333 -0.61666667 -0.6125 -0.60833333 -0.60416667 -0.6 -0.59583333 -0.59166667 -0.5875 -0.58333333 -0.57916667 -0.575 -0.57083333 -0.56666667 -0.5625 -0.55833333 -0.55416667 -0.55 -0.54583333 -0.54166667 -0.5375 -0.53333333 -0.52916667 -0.525 -0.52083333 -0.51666667 -0.5125 -0.50833333 -0.50416667 -0.5 -0.49583333 -0.49166667 -0.4875 -0.48333333 -0.47916667 -0.475 -0.47083333 -0.46666667 -0.4625 -0.45833333 -0.45416667 -0.45 -0.44583333 -0.44166667 -0.4375 -0.43333333 -0.42916667 -0.425 -0.42083333 -0.41666667 -0.4125 -0.40833333 -0.40416667 -0.4 -0.39583333 -0.39166667 -0.3875 -0.38333333 -0.37916667 -0.375 -0.37083333 -0.36666667 -0.3625 -0.35833333 -0.35416667 -0.35 -0.34583333 -0.34166667 -0.3375 -0.33333333 -0.32916667 -0.325 -0.32083333 -0.31666667 -0.3125 -0.30833333 -0.30416667 -0.3 -0.29583333 -0.29166667 -0.2875 -0.28333333 -0.27916667 -0.275 -0.27083333 -0.26666667 -0.2625 -0.25833333 -0.25416667 -0.25 -0.24583333 -0.24166667 -0.2375 -0.23333333 -0.22916667 -0.225 -0.22083333 -0.21666667 -0.2125 -0.20833333 -0.20416667 -0.2 -0.19583333 -0.19166667 -0.1875 -0.18333333 -0.17916667 -0.175 -0.17083333 -0.16666667 -0.1625 -0.15833333 -0.15416667 -0.15 -0.14583333 -0.14166667 -0.1375 -0.13333333 -0.12916667 -0.125 -0.12083333 -0.11666667 -0.1125 -0.10833333 -0.10416667 -0.1 -0.09583333 -0.09166667 -0.0875 -0.08333333 -0.07916667 -0.075 -0.07083333 -0.06666667 -0.0625 -0.05833333 -0.05416667 -0.05 -0.04583333 -0.04166667 -0.0375 -0.03333333 -0.02916667 -0.025 -0.02083333 -0.01666667 -0.0125 -0.00833333 -0.00416667 0 0 0 0 0 0
  arc A28 (-16.1526, -11.2836) -> (-15.1575, -11.9297) centre (0, 12.5) ccw
  line L65 (-26.1453, -0.1491) -> (-25.8803, -0.0209)
  line L66 (-27.8937, 20.5945) -> (-27.6109, 20.5125)
  spline S21 degree 5 poles (-27.8945, 4.4052) (-27.8946, 4.4052) (-27.8948, 4.4052) (-27.8951, 4.4051) (-27.8956, 4.4049) (-27.8963, 4.4047) (-27.8971, 4.4044) (-27.898, 4.4042) (-27.8991, 4.4038) (-27.9002, 4.4035) (-27.9015, 4.4031) (-27.9028, 4.4027) (-27.9043, 4.4022) (-27.9058, 4.4017) (-27.9075, 4.4012) (-27.9092, 4.4006) (-27.9111, 4.4) (-27.913, 4.3993) (-27.915, 4.3987) (-27.9172, 4.398) (-27.9194, 4.3972) (-27.9217, 4.3964) (-27.9241, 4.3956) (-27.9265, 4.3948) (-27.9291, 4.3939) (-27.9318, 4.393) (-27.9345, 4.392) (-27.9373, 4.391) (-27.9402, 4.39) (-27.9432, 4.3889) (-27.9462, 4.3879) (-27.9494, 4.3867) (-27.9526, 4.3856) (-27.9559, 4.3844) (-27.9593, 4.3831) (-27.9627, 4.3819) (-27.9662, 4.3806) (-27.9698, 4.3792) (-27.9735, 4.3778) (-27.9772, 4.3764) (-27.9811, 4.375) (-27.9849, 4.3735) (-27.9889, 4.372) (-27.9929, 4.3705) (-27.997, 4.3689) (-28.0012, 4.3673) (-28.0054, 4.3656) (-28.0097, 4.3639) (-28.0141, 4.3622) (-28.0185, 4.3605) (-28.023, 4.3587) (-28.0276, 4.3568) (-28.0322, 4.355) (-28.0369, 4.3531) (-28.0416, 4.3512) (-28.0464, 4.3492) (-28.0513, 4.3472) (-28.0562, 4.3452) (-28.0612, 4.3431) (-28.0663, 4.341) (-28.0714, 4.3389) (-28.0765, 4.3367) (-28.0818, 4.3345) (-28.087, 4.3323) (-28.0924, 4.33) (-28.0978, 4.3277) (-28.1032, 4.3253) (-28.1087, 4.323) (-28.1143, 4.3205) (-28.1199, 4.3181) (-28.1256, 4.3156) (-28.1313, 4.3131) (-28.1371, 4.3105) (-28.1429, 4.308) (-28.1488, 4.3053) (-28.1547, 4.3027) (-28.1607, 4.3) (-28.1667, 4.2973) (-28.1728, 4.2945) (-28.179, 4.2917) (-28.1851, 4.2889) (-28.1914, 4.286) (-28.1977, 4.2831) (-28.204, 4.2802) (-28.2104, 4.2773) (-28.2168, 4.2743) (-28.2233, 4.2712) (-28.2298, 4.2682) (-28.2363, 4.2651) (-28.2429, 4.2619) (-28.2496, 4.2588) (-28.2563, 4.2555) (-28.263, 4.2523) (-28.2698, 4.249) (-28.2767, 4.2457) (-28.2835, 4.2424) (-28.2905, 4.239) (-28.2974, 4.2356) (-28.3044, 4.2322) (-28.3115, 4.2287) (-28.3186, 4.2252) (-28.3257, 4.2216) (-28.3329, 4.218) (-28.3401, 4.2144) (-28.3473, 4.2108) (-28.3546, 4.2071) (-28.3619, 4.2034) (-28.3693, 4.1996) (-28.3767, 4.1958) (-28.3842, 4.192) (-28.3917, 4.1882) (-28.3992, 4.1843) (-28.4068, 4.1804) (-28.4144, 4.1764) (-28.422, 4.1724) (-28.4297, 4.1684) (-28.4374, 4.1643) (-28.4452, 4.1602) (-28.4529, 4.1561) (-28.4608, 4.152) (-28.4686, 4.1478) (-28.4765, 4.1435) (-28.4845, 4.1393) (-28.4924, 4.135) (-28.5004, 4.1307) (-28.5085, 4.1263) (-28.5165, 4.1219) (-28.5246, 4.1175) (-28.5328, 4.113) (-28.5409, 4.1085) (-28.5491, 4.104) (-28.5574, 4.0994) (-28.5657, 4.0948) (-28.574, 4.0902) (-28.5823, 4.0855) (-28.5907, 4.0808) (-28.5991, 4.0761) (-28.6075, 4.0713) (-28.616, 4.0665) (-28.6244, 4.0616) (-28.633, 4.0568) (-28.6415, 4.0519) (-28.6501, 4.0469) (-28.6587, 4.042) (-28.6674, 4.037) (-28.676, 4.0319) (-28.6847, 4.0268) (-28.6935, 4.0217) (-28.7022, 4.0166) (-28.711, 4.0114) (-28.7199, 4.0062) (-28.7287, 4.001) (-28.7376, 3.9957) (-28.7465, 3.9904) (-28.7554, 3.985) (-28.7644, 3.9797) (-28.7734, 3.9743) (-28.7824, 3.9688) (-28.7914, 3.9633) (-28.8005, 3.9578) (-28.8096, 3.9523) (-28.8187, 3.9467) (-28.8279, 3.9411) (-28.837, 3.9355) (-28.8462, 3.9298) (-28.8555, 3.9241) (-28.8647, 3.9183) (-28.874, 3.9126) (-28.8833, 3.9068) (-28.8926, 3.9009) (-28.902, 3.895) (-28.9113, 3.8891) (-28.9207, 3.8832) (-28.9302, 3.8772) (-28.9396, 3.8712) (-28.9491, 3.8652) (-28.9586, 3.8591) (-28.9681, 3.853) (-28.9776, 3.8468) (-28.9872, 3.8407) (-28.9968, 3.8344) (-29.0064, 3.8282) (-29.016, 3.8219) (-29.0257, 3.8156) (-29.0354, 3.8093) (-29.0451, 3.8029) (-29.0548, 3.7965) (-29.0646, 3.7901) (-29.0743, 3.7836) (-29.0841, 3.7771) (-29.0939, 3.7705) (-29.1037, 3.764) (-29.1136, 3.7574) (-29.1235, 3.7507) (-29.1334, 3.7441) (-29.1433, 3.7374) (-29.1532, 3.7306) (-29.1632, 3.7238) (-29.1731, 3.717) (-29.1831, 3.7102) (-29.1932, 3.7033) (-29.2032, 3.6964) (-29.2132, 3.6895) (-29.2233, 3.6825) (-29.2334, 3.6755) (-29.2435, 3.6685) (-29.2537, 3.6614) (-29.2638, 3.6543) (-29.274, 3.6472) (-29.2842, 3.64) (-29.2944, 3.6329) (-29.3046, 3.6256) (-29.3148, 3.6184) (-29.3251, 3.6111) (-29.3354, 3.6037) (-29.3457, 3.5964) (-29.356, 3.589) (-29.3663, 3.5816) (-29.3766, 3.5741) (-29.387, 3.5666) (-29.3974, 3.5591) (-29.4078, 3.5515) (-29.4182, 3.544) (-29.4286, 3.5363) (-29.4391, 3.5287) (-29.4495, 3.521) (-29.46, 3.5133) (-29.4705, 3.5055) (-29.481, 3.4978) (-29.4915, 3.4899) (-29.5021, 3.4821) (-29.5127, 3.4742) (-29.5232, 3.4663) (-29.5338, 3.4584) (-29.5444, 3.4504) (-29.555, 3.4424) (-29.5657, 3.4343) (-29.5763, 3.4263) (-29.587, 3.4182) (-29.5977, 3.41) (-29.6084, 3.4019) (-29.6169, 3.3953) (-29.6234, 3.3904) (-29.6276, 3.3871) (-29.6298, 3.3854) knots 0 0 0 0 0 0 0.00416667 0.00833333 0.0125 0.01666667 0.02083333 0.025 0.02916667 0.03333333 0.0375 0.04166667 0.04583333 0.05 0.05416667 0.05833333 0.0625 0.06666667 0.07083333 0.075 0.07916667 0.08333333 0.0875 0.09166667 0.09583333 0.1 0.10416667 0.10833333 0.1125 0.11666667 0.12083333 0.125 0.12916667 0.13333333 0.1375 0.14166667 0.14583333 0.15 0.15416667 0.15833333 0.1625 0.16666667 0.17083333 0.175 0.17916667 0.18333333 0.1875 0.19166667 0.19583333 0.2 0.20416667 0.20833333 0.2125 0.21666667 0.22083333 0.225 0.22916667 0.23333333 0.2375 0.24166667 0.24583333 0.25 0.25416667 0.25833333 0.2625 0.26666667 0.27083333 0.275 0.27916667 0.28333333 0.2875 0.29166667 0.29583333 0.3 0.30416667 0.30833333 0.3125 0.31666667 0.32083333 0.325 0.32916667 0.33333333 0.3375 0.34166667 0.34583333 0.35 0.35416667 0.35833333 0.3625 0.36666667 0.37083333 0.375 0.37916667 0.38333333 0.3875 0.39166667 0.39583333 0.4 0.40416667 0.40833333 0.4125 0.41666667 0.42083333 0.425 0.42916667 0.43333333 0.4375 0.44166667 0.44583333 0.45 0.45416667 0.45833333 0.4625 0.46666667 0.47083333 0.475 0.47916667 0.48333333 0.4875 0.49166667 0.49583333 0.5 0.50416667 0.50833333 0.5125 0.51666667 0.52083333 0.525 0.52916667 0.53333333 0.5375 0.54166667 0.54583333 0.55 0.55416667 0.55833333 0.5625 0.56666667 0.57083333 0.575 0.57916667 0.58333333 0.5875 0.59166667 0.59583333 0.6 0.60416667 0.60833333 0.6125 0.61666667 0.62083333 0.625 0.62916667 0.63333333 0.6375 0.64166667 0.64583333 0.65 0.65416667 0.65833333 0.6625 0.66666667 0.67083333 0.675 0.67916667 0.68333333 0.6875 0.69166667 0.69583333 0.7 0.70416667 0.70833333 0.7125 0.71666667 0.72083333 0.725 0.72916667 0.73333333 0.7375 0.74166667 0.74583333 0.75 0.75416667 0.75833333 0.7625 0.76666667 0.77083333 0.775 0.77916667 0.78333333 0.7875 0.79166667 0.79583333 0.8 0.80416667 0.80833333 0.8125 0.81666667 0.82083333 0.825 0.82916667 0.83333333 0.8375 0.84166667 0.84583333 0.85 0.85416667 0.85833333 0.8625 0.86666667 0.87083333 0.875 0.87916667 0.88333333 0.8875 0.89166667 0.89583333 0.9 0.90416667 0.90833333 0.9125 0.91666667 0.92083333 0.925 0.92916667 0.93333333 0.9375 0.94166667 0.94583333 0.95 0.95416667 0.95833333 0.9625 0.96666667 0.97083333 0.975 0.97916667 0.98333333 0.9875 0.99166667 0.99583333 1 1 1 1 1 1
  line L67 (-15.3128, -12.1799) -> (-15.3132, -12.1806)
  line L68 (-27.8945, 20.5948) -> (-27.8937, 20.5945)
  line L69 (-16.3184, -11.5278) -> (-16.318, -11.5271)
  line L70 (-28.587, 17.6345) -> (-28.2972, 17.5824)
  arc A29 (-18.5501, -9.4649) -> (-17.6281, -10.2115) centre (0, 12.5) ccw
  arc A30 (-15.9204, -14.0997) -> (-15.0758, -14.5873) centre (0, 12.5) ccw
  line L71 (-16.318, -11.5271) -> (-16.1526, -11.2836)